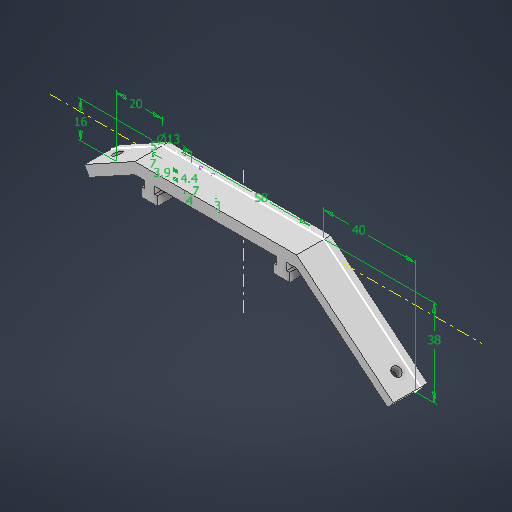
# Autodesk Inventor part: UnitreeGO2_railmount
Saved by Autodesk Inventor 2026.1 (Build 301233000, 233)
## iProperties
Created: 2026-01-16
Part Number: UnitreeGO2_railmount
Material: Generic
Document SubType Name: Modeling
Designer: aimot
Density: 1 g/cm^3
Appearance: Default
Author: aimot
Autodesk Inventor part; units mm, degrees
ref_plane "YZ Plane" through (0, 0, 0) normal (1, 0, 0) x (0, 1, 0)
ref_plane "XZ Plane" through (0, 0, 0) normal (0, 1, 0) x (-1, 0, 0)
ref_plane "XY Plane" through (0, 0, 0) normal (0, 0, 1) x (1, 0, 0)
sketch "Sketch2" plane through (0, 0, 0) normal (0, 0, 1) x (1, 0, 0)
  line L0 (-32.5, -3.1) -> (-25.5, -3.1)
  line L1 (-25.5, -3.1) -> (-25.5, -7)
  line L2 (-25.5, -7) -> (-32.5, -7)
  line L3 (-32.5, -7) -> (-32.5, -3.1)
  line L4 (-31.2, 0) -> (-26.8, 0)
  line L5 (-26.8, 0) -> (-26.8, -3.1)
  line L6 (-26.8, -3.1) -> (-31.2, -3.1)
  line L7 (-31.2, -3.1) -> (-31.2, 0)
  line L8 (-35.5, 0) -> (0, 0)
  line L9 (0, 5) -> (-35.5, 5)
  line L10 (-35.5, 5) -> (-35.5, 0)
  line L11 (-29, 6.5254) -> (-29, -10.3092) construction
  line L12 (0, -40.9051) -> (0, 14.4305) construction
  line L13 (32.5, -3.1) -> (25.5, -3.1)
  line L14 (25.5, -3.1) -> (25.5, -7)
  line L15 (25.5, -7) -> (32.5, -7)
  line L16 (32.5, -7) -> (32.5, -3.1)
  line L17 (31.2, 0) -> (26.8, 0)
  line L18 (26.8, 0) -> (26.8, -3.1)
  line L19 (26.8, -3.1) -> (31.2, -3.1)
  line L20 (31.2, -3.1) -> (31.2, 0)
  line L21 (35.5, 0) -> (0, 0)
  line L22 (0, 5) -> (35.5, 5)
  line L23 (35.5, 5) -> (35.5, 0)
  line L24 (29, 6.5254) -> (29, -10.3092) construction
  line L25 (-84.7245, 0) -> (105.0676, 0) construction
  line L26 (35.5, 5) -> (77.9544, -30.0249)
  line L27 (77.9544, -30.0249) -> (75.5, -33)
  line L28 (75.5, -33) -> (35.5, 0)
  line L29 (-35.5, 5) -> (35.5, 5)
  line L30 (35.5, 5) -> (35.5, -7)
  line L31 (35.5, -7) -> (-35.5, -7)
  line L32 (-35.5, -7) -> (-35.5, 5)
  line L33 (-35.5, 5) -> (-57.6113, -7.1612)
  line L34 (-57.6113, -7.1612) -> (-55.5, -11)
  line L35 (-55.5, -11) -> (-35.5, 0)
  line L36 (-21.5, -7) -> (-21.5, -4)
  line L37 (-21.5, -4) -> (0, -4)
  line L38 (21.5, -7) -> (21.5, -4)
  line L39 (21.5, -4) -> (0, -4)
  line L40 (-35.5, -7) -> (-48.2273, -7)
  line L41 (35.5, -7) -> (43.9848, -7)
  point P0 (-13.25, 5)
  point P1 (-18.25, 5)
  point P2 (29, -7)
  point P3 (32.5, -7)
  point P4 (-32.5, -7)
  point P5 (21.5, -7)
  dimension "d1" = 4.4
  dimension "d2" = 7
  dimension "d3" = 3.9
  dimension "d4" = 5
  dimension "d5" = 58
  dimension "d6" = 7
  dimension "d7" = 13
  dimension "d28" = 38
  dimension "d29" = 40
  dimension "d30" = 20
  dimension "d31" = 16
  dimension "d37" = 4
  dimension "d38" = 3
  constraints: 80 end point, 14 symmetric about line, 13 point on line, 9 parallel, 7 perpendicular, 6 horizontal, 1 collinear, 1 midpoint, 1 vertical, 2 other
  measures "d1" distance between parallel lines of L5 L7
  measures "d2" distance between parallel lines of L1 L3
  measures "d3" distance between parallel lines of L2 L0
  measures "d4" distance between parallel lines of L9 L8
  measures "d5" distance between parallel lines of L24 L11
  measures "d6" distance between parallel lines of L8 L2
  measures "d7" diameter of L10 L11
  measures "d28" vertical distance of L23.start L27.end
  measures "d29" horizontal distance of L27.end L23.start
  measures "d30" horizontal distance of L34.end L9.end
  measures "d31" vertical distance of L9.end L34.end
  measures "d37" distance between parallel lines of L36 L1
  measures "d38" distance between parallel lines of L37 L31
extrude "Extrusion1" add sketch "Sketch2" along normal blind 12 contours L0 L1 L2 L3 | L7 L4 L5 L0 | L8 L10 L9 L22 L23 L21 L17 L4 | L35 L34 L33 L10 | L17 L20 L13 L18 | L14 L13 L16 L15 | L26 L27 L28 L23
extrude "Extrusion3" add sketch "Sketch2" against normal blind 3 contours L3 L31 L32 L8 L7 L0 | L0 L1 L2 L3 | L7 L4 L5 L0 | L5 L8 L21 L18 L13 L14 L31 L38 L39 L37 L36 L1 L0 | L8 L10 L9 L22 L23 L21 L17 L4 | L40 L35 L32 | L35 L34 L33 L10 | L17 L20 L13 L18 | L14 L13 L16 L15 | L21 L30 L31 L16 L13 L20 | L26 L27 L28 L23 | L28 L41 L30
sketch "Sketch3" plane through (-57.6113, -7.1612, 12) normal (-0.4819, 0.8762, 0) x (0.8762, 0.4819, 0)
  circle A0 centre (8, 7.5) radius 2
  line L0 (0, 0) -> (0, 15) projected
  line L1 (25.235, 0) -> (0, 0) projected
  point P0 (53.9311, 12)
  dimension "d39" = 4
  dimension "d40" = 8
  dimension "d41" = 7.5
  constraints: 1 centre point
  measures "d39" diameter of A0
  measures "d40" distance from line of L0 A0.centre
  measures "d41" distance from line of L1 A0.centre
extrude "Extrusion4" cut sketch "Sketch3" against normal blind 10
sketch "Sketch4" plane through (35.5, 5, 12) normal (0.6364, 0.7714, 0) x (0.7714, -0.6364, 0)
  circle A0 centre (47.0375, 7.5) radius 2
  line L0 (55.0375, 15) -> (55.0375, 0) projected
  line L1 (0, 15) -> (55.0375, 15) projected
  point P0 (-24.2018, 12)
  dimension "d44" = 4
  dimension "d45" = 8
  dimension "d46" = 7.5
  constraints: 1 centre point
  measures "d44" diameter of A0
  measures "d45" distance from line of L0 A0.centre
  measures "d46" distance from line of L1 A0.centre
extrude "Extrusion5" cut sketch "Sketch4" against normal blind 10
body "Solid1"
